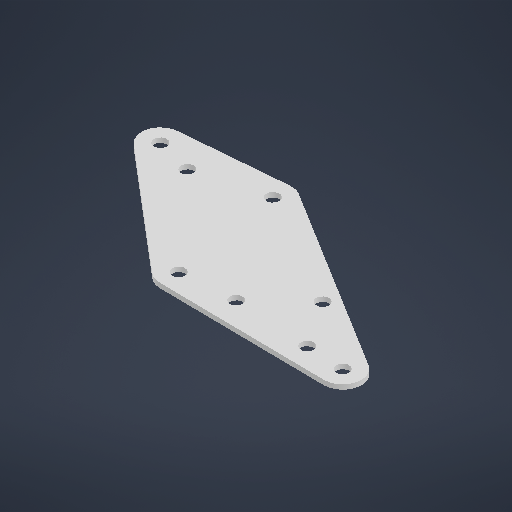
# Autodesk Inventor part: newsidepolytest
Saved by Autodesk Inventor 2025.2 (Build 292293000, 293)
## iProperties
Created: 2025-04-03
Part Number: newsidepolytest
Material: Generic
Document SubType Name: Modeling
Designer: Jahan
Density: 1 g/cm^3
Appearance: Default
Author: Jahan
Autodesk Inventor part; units mm, degrees
ref_plane "YZ Plane" through (0, 0, 0) normal (1, 0, 0) x (0, 1, 0)
ref_plane "XZ Plane" through (0, 0, 0) normal (0, 1, 0) x (-1, 0, 0)
ref_plane "XY Plane" through (0, 0, 0) normal (0, 0, 1) x (1, 0, 0)
sketch "Sketch1" plane through (0, 0, 0) normal (0, 1, 0) x (-1, 0, 0)
  circle A0 centre (-15.276282, 11.719172) radius 2.1844
  circle A1 centre (46.199401, -4.186485) radius 2.1844
  circle A2 centre (-0.285427, 25.848806) radius 2.1844
  circle A3 centre (-25.645908, 27.265134) radius 2.1844
  circle A4 centre (17.648799, 27.264625) radius 2.1844
  circle A5 centre (23.589254, -10.368908) radius 2.1844
  circle A6 centre (-38.326149, 27.973298) radius 2.1844
  circle A7 centre (58.494539, -7.367616) radius 2.1844
  circle A8 centre (-38.326149, 27.973298) radius 6.35
  circle A9 centre (23.589254, -10.368908) radius 6.35
  line L0 (-41.66936, 22.574646) -> (20.246043, -15.76756)
  circle A10 centre (17.648799, 27.264625) radius 6.35
  line L1 (17.729187, 33.614116) -> (-38.245761, 34.322789)
  circle A11 centre (46.199401, -4.186485) radius 6.35
  circle A12 centre (58.494539, -7.367616) radius 6.35
  line L2 (21.755399, 32.108005) -> (62.601139, -2.524235)
  line L3 (22.350491, 31.532714) -> (50.901093, 0.081604)
  line L4 (24.133244, -16.695564) -> (59.038529, -13.694272)
  line L5 (17.648799, 27.264625) -> (23.589254, -10.368908)
  line L6 (23.589254, -10.368908) -> (36.13393, -8.38873)
  line L7 (24.579343, -16.641246) -> (37.124019, -14.661068)
  line L8 (48.645825, -10.046307) -> (38.580353, -14.248552)
  arc A13 (37.124019, -14.661068) -> (38.580353, -14.248552) centre (36.13393, -8.38873) ccw
  point P0 (0, 0)
  dimension "d0" = 12.7
  dimension "d1" = 12.7
  dimension "d2" = 12.7
  dimension "d3" = 12.7
  dimension "d4" = 12.7
  dimension "d5" = 12.7
  dimension "d7" = 6.35
  constraints: 18 end point, 14 centre point, 14 point on circle, 12 tangent, 5 coincident, 1 perpendicular
  measures "d0" diameter of A8
  measures "d1" diameter of A9
  measures "d2" diameter of A10
  measures "d3" diameter of A11
  measures "d4" diameter of A12
  measures "d5" distance of L5.end L6.end
  measures "d7" radius of A13
extrude "Extrusion1" add sketch "Sketch1" along normal blind 1.5875 contours A5 L6 A9 L5 | A5 L5 A9 L6 | A9 L5 A10 L3 A11 L8 A13 L7 | A9 L0 A8 L1 A10 L5 | A10 | L7 A13 L8 A11 A12 L4 A9 | A8 | A12 | L2 A12 A11 L3 A10 | A11
body "Solid1"
